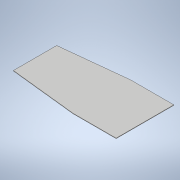
# Autodesk Inventor part: frontfloor
Saved by Autodesk Inventor 2021 (Build 250183000, 183)
## iProperties
Created: 2020-10-26
Part Number: frontfloor
Material: Generic
Document SubType Name: Modeling
Designer: mackeycj
Density: 1 g/cm^3
Appearance: Default
Author: mackeycj
Autodesk Inventor part; units mm, degrees
ref_plane "YZ Plane" through (0, 0, 0) normal (1, 0, 0) x (0, 1, 0)
ref_plane "XZ Plane" through (0, 0, 0) normal (0, 1, 0) x (-1, 0, 0)
ref_plane "XY Plane" through (0, 0, 0) normal (0, 0, 1) x (1, 0, 0)
sketch "Sketch1" plane through (0, 0, 0) normal (0, 1, 0) x (-1, 0, 0)
  line L0 (0, 0) -> (0, 203.2)
  line L1 (0, 203.2) -> (304.8, 203.2)
  line L2 (0, 0) -> (774.7, 0)
  line L3 (0, 0) -> (0, -203.2)
  line L4 (0, -203.2) -> (304.8, -203.2)
  line L5 (774.7, 0) -> (774.7, -152.4)
  line L6 (774.7, -152.4) -> (774.7, 0)
  line L7 (774.7, 0) -> (774.7, 152.4)
  line L8 (774.7, 152.4) -> (304.8, 203.2)
  line L9 (774.7, -152.4) -> (304.8, -203.2)
  dimension "d0" = 203.2
  dimension "d1" = 304.8
  dimension "d2" = 774.7
  dimension "d3" = 203.2
  dimension "d4" = 304.8
  dimension "d5" = 152.4
  dimension "d6" = 152.4
  constraints: 20 end point, 3 perpendicular, 3 vertical, 1 collinear, 1 horizontal
  measures "d0" distance of L0.start L0.end
  measures "d1" distance of L0.end L1.end
  measures "d2" distance of L0.start L2.end
  measures "d3" distance of L0.start L3.end
  measures "d4" distance of L3.end L4.end
  measures "d5" distance of L2.end L5.end
  measures "d6" distance of L2.end L7.end
extrude "Extrusion1" add sketch "Sketch1" along normal blind 3.175
body "Solid1"
